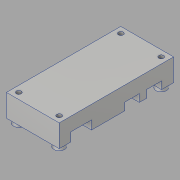
# Autodesk Inventor part: Heat Block for Pi
Saved by Autodesk Inventor 2017 (Build 210142000, 142)
## iProperties
Created: 2017-02-16
Part Number: Heat Block for Pi
Material: Aluminum 6061
Document SubType Name: Modeling
Designer: qupec
Density: 2.7 g/cm^3
Appearance: Aluminum - Flat
Author: qupec
Autodesk Inventor part; units mm, degrees
ref_plane "YZ Plane" through (0, 0, 0) normal (1, 0, 0) x (0, 1, 0)
ref_plane "XZ Plane" through (0, 0, 0) normal (0, 1, 0) x (-1, 0, 0)
ref_plane "XY Plane" through (0, 0, 0) normal (0, 0, 1) x (1, 0, 0)
sketch "Sketch1" plane through (0, 0, 0) normal (0, 1, 0) x (-1, 0, 0)
  line L0 (15, 32.5) -> (-15, 32.5)
  line L1 (-15, 32.5) -> (-15, -32.5)
  line L2 (-15, -32.5) -> (15, -32.5)
  line L3 (15, -32.5) -> (15, 32.5)
  point P0 (0, 0)
  dimension "d0" = 65
  dimension "d1" = 30
  dimension "d2" = 15
  dimension "d3" = 32.5
  constraints: 8 end point, 2 parallel, 1 horizontal, 1 perpendicular
  measures "d0" distance between parallel lines of L2 L0
  measures "d1" distance between parallel lines of L1 L3
  measures "d2" distance from line of point (0, 0) L1
  measures "d3" distance from line of point (0, 0) L0
extrude "Extrusion1" add sketch "Sketch1" along normal blind 12.7
sketch "Sketch2" plane through (0, 0, 0) normal (0, -1, 0) x (1, 0, 0)
  line L0 (8.07, 8.904) -> (-4.13, 8.904)
  line L1 (-4.13, 8.904) -> (-4.13, -3.296)
  line L2 (-4.13, -3.296) -> (8.07, -3.296)
  line L3 (8.07, -3.296) -> (8.07, 8.904)
  line L4 (-15, 32.5) -> (15, 32.5) projected
  line L5 (15, 32.5) -> (15, -32.5) projected
  point P0 (0, 0)
  dimension "d6" = 12.2
  dimension "d7" = 12.2
  dimension "d8" = 23.596
  dimension "d9" = 6.93
  constraints: 8 end point, 2 parallel, 1 horizontal, 1 perpendicular
  measures "d6" distance between parallel lines of L2 L0
  measures "d7" distance between parallel lines of L1 L3
  measures "d8" distance between parallel lines of L4 L0
  measures "d9" distance between parallel lines of L5 L3
extrude "Extrusion2" add sketch "Sketch2" along normal blind 1.17
sketch "Sketch3" plane through (0, 0, 0) normal (0, -1, 0) x (1, 0, 0)
  line L0 (15, 32.5) -> (15, -32.5) projected
  line L1 (15, 25.85) -> (7.4, 25.85)
  line L2 (7.4, 25.85) -> (7.4, 14.15)
  line L3 (7.4, 14.15) -> (15, 14.15)
  line L4 (15, 14.15) -> (15, 25.85)
  line L5 (-15, 32.5) -> (15, 32.5) projected
  point P0 (0, 0)
  dimension "d12" = 7.6
  dimension "d13" = 11.7
  dimension "d14" = 6.65
  constraints: 8 end point, 2 parallel, 1 horizontal, 1 perpendicular, 1 point on line
  measures "d12" distance of L1.start L1.end
  measures "d13" distance between parallel lines of L3 L1
  measures "d14" distance between parallel lines of L5 L1
extrude "Extrusion3" cut sketch "Sketch3" against normal blind 5
sketch "Sketch4" plane through (0, 0, 0) normal (0, -1, 0) x (1, 0, 0)
  line L0 (15, 14.15) -> (15, -32.5) projected
  line L1 (15, -4.75) -> (10.3, -4.75)
  line L2 (10.3, -4.75) -> (10.3, -13.05)
  line L3 (10.3, -13.05) -> (15, -13.05)
  line L4 (15, -13.05) -> (15, -4.75)
  line L5 (-15, 32.5) -> (15, 32.5) projected
  point P0 (0, 0)
  dimension "d17" = 4.7
  dimension "d18" = 8.3
  dimension "d19" = 37.25
  constraints: 8 end point, 2 parallel, 1 horizontal, 1 perpendicular, 1 point on line
  measures "d17" distance between parallel lines of L2 L0
  measures "d18" distance between parallel lines of L3 L1
  measures "d19" distance between parallel lines of L5 L1
extrude "Extrusion4" cut sketch "Sketch4" against normal blind 4.3
sketch "Sketch5" plane through (0, 0, 0) normal (0, -1, 0) x (1, 0, 0)
  line L0 (15, -13.05) -> (15, -32.5) projected
  line L1 (15, -17.35) -> (10.3, -17.35)
  line L2 (10.3, -17.35) -> (10.3, -25.65)
  line L3 (10.3, -25.65) -> (15, -25.65)
  line L4 (15, -25.65) -> (15, -17.35)
  line L5 (15, -32.5) -> (-15, -32.5) projected
  point P0 (0, 0)
  dimension "d22" = 4.7
  dimension "d23" = 8.3
  dimension "d24" = 6.85
  constraints: 8 end point, 2 parallel, 1 horizontal, 1 perpendicular, 1 point on line
  measures "d22" distance of L3.end L2.end
  measures "d23" distance between parallel lines of L3 L1
  measures "d24" distance between parallel lines of L5 L3
extrude "Extrusion5" cut sketch "Sketch5" against normal blind 4.3
sketch "Sketch6" plane through (0, 0, 0) normal (0, -1, 0) x (1, 0, 0)
  circle A0 centre (11.5, 29) radius 3
  circle A1 centre (-11.5, 29) radius 3
  circle A2 centre (-11.5, -29) radius 3
  circle A3 centre (11.5, -29) radius 3
  line L0 (15, -32.5) -> (-15, -32.5) projected
  line L1 (-15, -32.5) -> (-15, 32.5) projected
  line L2 (-15, 32.5) -> (15, 32.5) projected
  point P0 (0, 0)
  dimension "d27" = 6
  dimension "d28" = 6
  dimension "d29" = 6
  dimension "d30" = 6
  dimension "d31" = 0
  dimension "d32" = 23
  dimension "d33" = 58
  dimension "d34" = 3.5
  dimension "d35" = 23
  dimension "d37" = 0
  dimension "d38" = 3.5
  dimension "d42" = 3.5
  constraints: 4 centre point
  measures "d27" diameter of A0
  measures "d28" diameter of A3
  measures "d29" diameter of A2
  measures "d30" diameter of A1
  measures "d31" vertical distance of A2.centre A3.centre
  measures "d32" distance of A1.centre A0.centre
  measures "d33" distance of A2.centre A1.centre
  measures "d34" distance from line of L0 A2.centre
  measures "d35" distance of A3.centre A2.centre
  measures "d37" horizontal distance of A3.centre A0.centre
  measures "d38" distance from line of L1 A2.centre
  measures "d42" distance from line of L2 A0.centre
extrude "Extrusion6" add sketch "Sketch6" along normal blind 2.42
sketch "Sketch7" plane through (11.5, -2.42, 29) normal (0, -1, 0) x (1, 0, 0)
  circle A0 centre (0, 0) radius 3 projected
  circle A1 centre (0, -58) radius 3 projected
  circle A2 centre (-23, -58) radius 3 projected
  circle A3 centre (-23, 0) radius 3 projected
  point P0 (-11.5, -29)
  constraints: 4 coincident
hole "Hole1" at (11.5, -2.42, 29) at (-11.5, -2.42, 29) at (-11.5, -2.42, -29) at (11.5, -2.42, -29) direction (0, 1, 0) diameter 2.75 depth 25.4 tip angle 118
sketch "Sketch8" plane through (0, 0, 0) normal (0, -1, 0) x (1, 0, 0)
  line L0 (15, -32.5) -> (-15, -32.5) projected
  line L1 (8.255, -32.5) -> (-8.255, -32.5)
  line L2 (-8.255, -32.5) -> (-8.255, -27.166)
  line L3 (-8.255, -27.166) -> (8.255, -27.166)
  line L4 (8.255, -27.166) -> (8.255, -32.5)
  point P0 (0, 0)
  point P1 (0, 0)
  dimension "d50" = 5.334
  dimension "d51" = 16.51
  dimension "d52" = 8.255
  constraints: 8 end point, 2 parallel, 1 coincident, 1 horizontal, 1 perpendicular, 1 point on line
  measures "d50" distance between parallel lines of L0 L3
  measures "d51" distance between parallel lines of L2 L4
  measures "d52" distance from line of L2 point (0, 0)
extrude "Extrusion7" cut sketch "Sketch8" against normal blind 2.032
sketch "Sketch9" plane through (0, 0, 0) normal (0, -1, 0) x (1, 0, 0)
  line L0 (4.228, 30.9) -> (-7.722, 30.9)
  line L1 (-7.722, 30.9) -> (-7.722, 19.5)
  line L2 (-7.722, 19.5) -> (4.228, 19.5)
  line L3 (4.228, 19.5) -> (4.228, 30.9)
  line L4 (-15, 32.5) -> (15, 32.5) projected
  line L5 (-15, -32.5) -> (-15, 32.5) projected
  line L6 (15, 32.5) -> (15, 25.85) projected
  point P0 (0, 0)
  dimension "d56" = 1.6
  dimension "d57" = 11.4
  dimension "d58" = 11.95
  dimension "d60" = 10.772
  constraints: 8 end point, 2 parallel, 1 horizontal, 1 perpendicular
  measures "d56" distance between parallel lines of L0 L4
  measures "d57" distance of L2.end L0.start
  measures "d58" distance between parallel lines of L1 L3
  measures "d60" distance between parallel lines of L6 L3
extrude "Extrusion9" add sketch "Sketch9" along normal blind 0.1111
equation "\"d2\" = 0.5 * d1"
equation "\"d3\" = 0.5 * d0"
equation "\"d6\" = d7"
equation "\"d28\" = d27"
equation "\"d29\" = d27"
equation "\"d30\" = d27"
equation "\"d35\" = d32"
equation "\"d52\" = 0.5 * d51"
body "Solid1"
